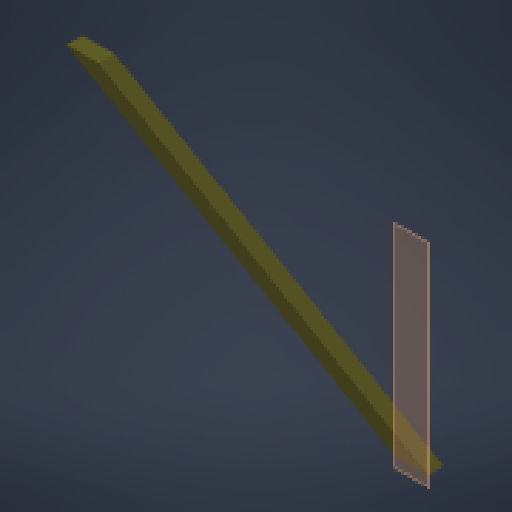
# Autodesk Inventor part: 2x4x(24x43)
Saved by Autodesk Inventor 2027 (Build 310192000, 192)
## iProperties
Created: 2026-05-29
Part Number: 2x4x(24x43)
Material: Generic
Document SubType Name: Modeling
Designer: lucas
Density: 1 g/cm^3
Appearance: Default
Author: lucas
Autodesk Inventor part; units mm, degrees
ref_plane "YZ Plane" through (0, 0, 0) normal (1, 0, 0) x (0, 1, 0)
ref_plane "XZ Plane" through (0, 0, 0) normal (0, 1, 0) x (-1, 0, 0)
ref_plane "XY Plane" through (0, 0, 0) normal (0, 0, 1) x (1, 0, 0)
ref_plane "Work Plane1" through (0, 0, 0) normal (0, 0, 1) x (1, 0, 0)
sketch "Sketch1" plane through (0, 0, 0) normal (0, 0, 1) x (1, 0, 0)
  line L0 (-1092.2, 304.8) -> (-1041.4, 304.8) projected
  line L1 (-50.8, -245.3386) -> (50.8, -304.8) projected
  line L2 (-1041.4, 304.8) -> (1524, 304.8) projected
  line L3 (-990.8062, 304.8) -> (-1092.2, 304.8)
  line L4 (-990.8062, 304.8) -> (-1092.2, 304.8)
  line L5 (-990.8062, 304.8) -> (-1092.2, 304.8)
  line L6 (50.8, -304.8) -> (-227.6342, -141.8464)
  line L7 (-227.6342, -141.8464) -> (-990.8062, 304.8)
  line L8 (-990.8062, 304.8) -> (-1092.2, 304.8)
  line L9 (-1092.2, 304.8) -> (-50.5938, -304.8)
  line L10 (50.8, -304.8) -> (-50.5938, -304.8)
  point P0 (-905.0447, 254.6081)
  point P1 (-930.9134, 210.407)
  point P2 (-162.6995, -179.8494)
  constraints: 16 end point, 4 collinear, 3 point on line, 1 horizontal, 1 parallel, 2 other
extrude "Extrusion1" add sketch "Sketch1" against normal blind 50.8
body "Solid1"
